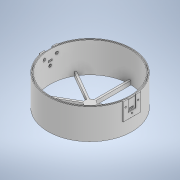
# Autodesk Inventor part: Base
Saved by Autodesk Inventor 2020.2 (Build 242310000, 310)
## iProperties
Created: 2020-04-11
Part Number: Base
Material: Generic
Document SubType Name: Modeling
Designer: Josiah
Density: 1 g/cm^3
Appearance: Default
Author: Josiah
Autodesk Inventor part; units mm, degrees
note: some values were not read from the file. Chosen so that the rebuilt part matches the saved one: second side of "Extrusion8".
ref_plane "YZ Plane" through (0, 0, 0) normal (1, 0, 0) x (0, 1, 0)
ref_plane "XZ Plane" through (0, 0, 0) normal (0, 1, 0) x (-1, 0, 0)
sketch "Sketch2" plane through (0, 0, 0) normal (0, 1, 0) x (-1, 0, 0)
  circle A0 centre (0, 0) radius 107.5
  circle A1 centre (0, 0) radius 102.5 construction
  circle A2 centre (0, 0) radius 12.5 construction
  line L0 (2.5, -12.2474) -> (2.5, -102.4695)
  line L1 (-2.5, -12.2474) -> (-2.5, -102.4695)
  arc A3 (-9.3566, -8.2888) -> (-2.5, -12.2474) centre (0, 0) ccw
  line L2 (0, 0) -> (-9.3566, -8.2888) construction
  line L3 (0, 0) -> (-2.5, -12.2474) construction
  line L4 (0, 0) -> (0, -103.4807) construction
  arc A4 (-87.4912, -53.3998) -> (-2.5, -102.4695) centre (0, 0) ccw
  line L5 (0, 0) -> (-87.4912, -53.3998) construction
  line L6 (0, 0) -> (-2.5, -102.4695) construction
  line L7 (11.8566, -3.9587) -> (89.9912, -49.0697)
  line L8 (9.3566, -8.2888) -> (87.4912, -53.3998)
  arc A5 (2.5, -102.4695) -> (87.4912, -53.3998) centre (0, 0) ccw
  arc A6 (2.5, -12.2474) -> (9.3566, -8.2888) centre (0, 0) ccw
  line L9 (9.3566, 8.2888) -> (87.4912, 53.3998)
  line L10 (11.8566, 3.9587) -> (89.9912, 49.0697)
  arc A7 (89.9912, -49.0697) -> (89.9912, 49.0697) centre (0, 0) ccw
  arc A8 (11.8566, -3.9587) -> (11.8566, 3.9587) centre (0, 0) ccw
  line L11 (-2.5, 12.2474) -> (-2.5, 102.4695)
  line L12 (2.5, 12.2474) -> (2.5, 102.4695)
  arc A9 (87.4912, 53.3998) -> (2.5, 102.4695) centre (0, 0) ccw
  arc A10 (9.3566, 8.2888) -> (2.5, 12.2474) centre (0, 0) ccw
  line L13 (-11.8566, 3.9587) -> (-89.9912, 49.0697)
  line L14 (-9.3566, 8.2888) -> (-87.4912, 53.3998)
  arc A11 (-2.5, 102.4695) -> (-87.4912, 53.3998) centre (0, 0) ccw
  arc A12 (-2.5, 12.2474) -> (-9.3566, 8.2888) centre (0, 0) ccw
  line L15 (-9.3566, -8.2888) -> (-87.4912, -53.3998)
  line L16 (-11.8566, -3.9587) -> (-89.9912, -49.0697)
  arc A13 (-89.9912, 49.0697) -> (-89.9912, -49.0697) centre (0, 0) ccw
  arc A14 (-11.8566, 3.9587) -> (-11.8566, -3.9587) centre (0, 0) ccw
  line L17 (0, 0) -> (2.5, 102.4695) construction
  line L18 (87.4912, 53.3998) -> (0, 0) construction
  point P0 (-89.9912, 49.0697)
  point P1 (-2.5, 12.2474)
  point P2 (-87.4912, -53.3998)
  point P3 (-9.3566, -8.2888)
  point P4 (89.9912, -49.0697)
  point P5 (11.8566, -3.9587)
  point P6 (2.5, -102.4695)
  dimension "wallThickness" = 5
  dimension "outerRadius" = 215
  dimension "innerRadius" = 25
  dimension "spokeHeight" = 5
  dimension "d15" = 2.5
  dimension "spokes" = 36.926
  dimension "d34" = 57.205
  dimension "d37" = 360
  constraints: 38 end point, 29 point on circle, 15 centre point, 6 coincident, 1 parallel, 1 point on line, 1 vertical, 73 other
  measures "wallThickness" radial gap between concentric circles of A0 A1
  measures "outerRadius" diameter of A0
  measures "innerRadius" diameter of A2
  measures "spokeHeight" distance between parallel lines of L1 L0
  measures "d15" distance from line of L1 point (0, 0)
  measures "spokes" angle of L2 L3
  measures "d34" angle of L5 L6
extrude "Extrusion1" add sketch "Sketch2" along normal blind 10
sketch "Sketch3" plane through (0, 10, 0) normal (0, 1, 0) x (1, 0, 0)
  circle A0 centre (0, 0) radius 107.5
  circle A1 centre (0, 0) radius 102.5
  dimension "d43" = 215
  dimension "d44" = 205
  constraints: 2 centre point, 2 coincident
  measures "d43" diameter of A0
  measures "d44" diameter of A1
extrude "Extrusion2" add sketch "Sketch3" along normal blind 67.5
ref_plane "Work Plane2" through (107.5, 0, 0) normal (1, 0, 0) x (0, 1, 0)
sketch "Sketch9" plane through (107.5, 0, 0) normal (1, 0, 0) x (0, 1, 0)
  line L0 (77.5, 102.5) -> (77.5, -102.5) projected
  line L1 (77.5, -22.5) -> (32.5, -22.5)
  line L2 (32.5, -22.5) -> (32.5, 22.5)
  line L3 (32.5, 22.5) -> (77.5, 22.5)
  line L4 (77.5, 22.5) -> (77.5, -22.5)
  line L5 (0, 0) -> (77.5, 0) construction
  point P0 (77.5, -22.5)
  point P1 (77.5, 22.5)
  dimension "d109" = 0
  dimension "d110" = 45
  dimension "d111" = 22.5
  dimension "d112" = 45
  constraints: 10 end point, 2 parallel, 2 perpendicular, 1 horizontal, 1 midpoint
  measures "d109" distance between parallel lines of L4 L0
  measures "d110" distance of L1.end L2.end
  measures "d111" distance between parallel lines of L5 L1
  measures "d112" distance of L1.start L1.end
extrude "Extrusion8" add sketch "Sketch9" against normal blind 3
sketch "Sketch5" plane through (107.5, 0, 0) normal (1, 0, 0) x (0, 1, 0)
  line L0 (77.5, -10) -> (47.5, -10)
  line L1 (47.5, -10) -> (47.5, 10)
  line L2 (47.5, 10) -> (77.5, 10)
  line L3 (77.5, 10) -> (77.5, -10)
  line L4 (77.5, -107.5) -> (77.5, 107.5) projected
  point P0 (0, 0)
  dimension "d60" = 20
  dimension "d61" = 0
  dimension "d62" = 30
  dimension "d63" = 10
  constraints: 8 end point, 2 parallel, 1 horizontal, 1 perpendicular
  measures "d60" distance between parallel lines of L2 L0
  measures "d61" distance between parallel lines of L4 L3
  measures "d62" distance of L0.start L0.end
  measures "d63" distance from line of point (0, 0) L0
extrude "Extrusion4" cut sketch "Sketch5" against normal blind 2 and the other way blind 2
sketch "Sketch7" plane through (0, 77.5, 0) normal (0, 1, 0) x (1, 0, 0)
  circle A0 centre (0, 0) radius 104.1167
  circle A1 centre (0, 0) radius 105.8833
  dimension "d84" = 208.2333
  dimension "d85" = 211.7667
  constraints: 2 centre point, 2 coincident
  measures "d84" diameter of A0
  measures "d85" diameter of A1
extrude "Extrusion6" cut sketch "Sketch7" against normal blind 4
ref_plane "Work Plane4" through (102.5, 0, 0) normal (1, 0, 0) x (0, 1, 0)
sketch "Sketch10" plane through (107.5, 0, 0) normal (1, 0, 0) x (0, 0, -1)
  line L0 (5, 50.5) -> (-5, 50.5)
  line L1 (-5, 50.5) -> (-5, 54.5)
  line L2 (-5, 54.5) -> (5, 54.5)
  line L3 (5, 54.5) -> (5, 50.5)
  line L4 (10, 47.5) -> (-10, 47.5) projected
  line L5 (10, 77.5) -> (10, 47.5) projected
  line L6 (-10, 47.5) -> (-10, 77.5) projected
  circle A0 centre (16, 62.5) radius 2
  line L7 (0, 47.5) -> (0, 77.5) construction
  line L8 (104.1167, 77.5) -> (-104.1167, 77.5) construction
  circle A1 centre (-16, 62.5) radius 2
  circle A2 centre (0, 41.5) radius 2
  point P0 (0, 0)
  dimension "d122" = 3
  dimension "d123" = 20
  dimension "d124" = 30
  dimension "d126" = 5
  dimension "d127" = 10
  dimension "d128" = 4
  dimension "d129" = 4
  dimension "d130" = 6
  dimension "d131" = 15
  dimension "d132" = 4
  dimension "d133" = 6
  dimension "d134" = 10
  constraints: 10 end point, 3 centre point, 2 midpoint, 2 parallel, 1 horizontal, 1 perpendicular, 1 symmetric about line, 1 other
  measures "d122" distance between parallel lines of L0 L4
  measures "d123" distance of L4.start L4.end
  measures "d124" distance of L5.start L4.start
  measures "d126" distance between parallel lines of L6 L1
  measures "d127" distance of L1.end L2.end
  measures "d128" distance between parallel lines of L0 L2
  measures "d129" diameter of A0
  measures "d130" distance from line of L5 A0.centre
  measures "d131" distance from line of L4 A0.centre
  measures "d132" diameter of A2
  measures "d133" distance from line of L4 A2.centre
  measures "d134" distance from line of L5 A2.centre
extrude "Extrusion9" cut sketch "Sketch10" against normal blind 15
sketch "Sketch11" plane through (0, 77.5, 0) normal (0, 1, 0) x (1, 0, 0)
  line L0 (107.5, -10) -> (105.5, -10) projected
  line L1 (107.5, -10) -> (104.1167, -10)
  line L2 (104.1167, -10) -> (104.1167, 10)
  line L3 (104.1167, 10) -> (107.5, 10)
  line L4 (107.5, 10) -> (107.5, -10)
  circle A0 centre (0, 0) radius 104.1167 projected
  point P0 (105.5, -10)
  dimension "d141" = 0
  dimension "d142" = 20
  constraints: 8 end point, 2 parallel, 1 horizontal, 1 perpendicular
  measures "d141" distance edge to line of A0 L2
  measures "d142" distance between parallel lines of L0 L3
extrude "Extrusion10" cut sketch "Sketch11" against normal up to surface (4 mm away) contours L0 L1 L2 L3 L4
sketch "Sketch12" plane through (102.5, 0, 0) normal (1, 0, 0) x (0, 1, 0)
  line L0 (38, -2.0207) -> (38, 2.0207)
  line L1 (38, 2.0207) -> (41.5, 4.0415)
  line L2 (41.5, 4.0415) -> (45, 2.0207)
  line L3 (45, 2.0207) -> (45, -2.0207)
  line L4 (45, -2.0207) -> (41.5, -4.0415)
  line L5 (41.5, -4.0415) -> (38, -2.0207)
  line L6 (59, -18.0207) -> (59, -13.9793)
  line L7 (59, -13.9793) -> (62.5, -11.9585)
  line L8 (62.5, -11.9585) -> (66, -13.9793)
  line L9 (66, -13.9793) -> (66, -18.0207)
  line L10 (66, -18.0207) -> (62.5, -20.0415)
  line L11 (62.5, -20.0415) -> (59, -18.0207)
  line L12 (77.5, 102.5) -> (77.5, -102.5) construction
  line L13 (77.5, 0) -> (47.5, 0) construction
  line L14 (47.5, -10) -> (47.5, 10) construction
  line L15 (59, 18.0207) -> (59, 13.9793)
  line L16 (59, 13.9793) -> (62.5, 11.9585)
  line L17 (62.5, 11.9585) -> (66, 13.9793)
  line L18 (66, 13.9793) -> (66, 18.0207)
  line L19 (66, 18.0207) -> (62.5, 20.0415)
  line L20 (62.5, 20.0415) -> (59, 18.0207)
  line L21 (73.5, -10) -> (47.5, -10) construction
  line L22 (47.5, 10) -> (73.5, 10) construction
  point P0 (0, 0)
  point P1 (41.5, 0)
  point P2 (62.5, -16)
  point P3 (62.5, 16)
  dimension "d145" = 6
  dimension "d146" = 15
  dimension "d147" = 7
  dimension "d148" = 7
  dimension "d149" = 6
  dimension "d150" = 10
  dimension "d151" = 0
  dimension "d152" = 0
  constraints: 38 end point, 7 symmetric about line, 2 midpoint, 26 other
  measures "d145" distance from line of L21 point (62.5, -16)
  measures "d146" distance from line of L14 point (62.5, -16)
  measures "d147" distance between parallel lines of L11 L8
  measures "d148" distance between parallel lines of L1 L4
  measures "d149" distance from line of L14 point (41.5, 0)
  measures "d150" distance from line of L21 point (41.5, 0)
  measures "d151" horizontal distance of L1.end point (41.5, 0)
  measures "d152" horizontal distance of point (62.5, -16) L7.end
extrude "Extrusion11" cut sketch "Sketch12" along normal blind 3 and the other way blind 5
pattern_circular "Circular Pattern2" count 2 over 360 about axis through (0, 0, 0) along (0, 1, 0) of "Extrusion8", "Extrusion9", "Extrusion4", "Extrusion10", "Extrusion11"
equation "\"spokeHeight\" = wallThickness"
equation "\"d15\" = 0.5 * spokeHeight"
equation "\"d43\" = outerRadius"
equation "\"d44\" = outerRadius - 2 * wallThickness"
body "Solid1"
